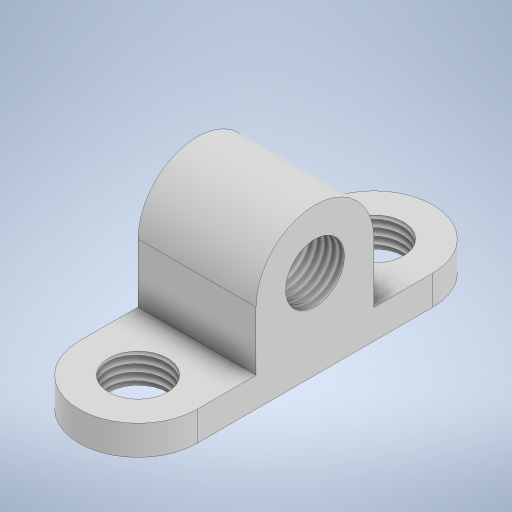
# Autodesk Inventor part: Tarea 1 Lab Dinamica
Saved by Autodesk Inventor 2024 (Build 280153000, 153)
## iProperties
Created: 2024-01-23
Part Number: Tarea 1 Lab Dinamica
Material: Genérico
Document SubType Name: Modeling
Designer: pazjo
Density: 1 g/cm^3
Appearance: Valor por defecto
Author: pazjo
Autodesk Inventor part; units mm, degrees
ref_plane "YZ Plane" through (0, 0, 0) normal (1, 0, 0) x (0, 1, 0)
ref_plane "XZ Plane" through (0, 0, 0) normal (0, 1, 0) x (-1, 0, 0)
ref_plane "XY Plane" through (0, 0, 0) normal (0, 0, 1) x (1, 0, 0)
sketch "Boceto1" plane through (0, 0, 0) normal (0, 1, 0) x (-1, 0, 0)
  line L0 (-20, 20) -> (-20, -20)
  line L1 (20, -20) -> (20, 20)
  arc A0 (20, 40) -> (-20, 40) centre (0, 40) ccw
  arc A1 (-20, -40) -> (20, -40) centre (0, -40) ccw
  circle A2 centre (0, -40) radius 10
  line L2 (20, 20) -> (20, 40)
  line L3 (-20, 20) -> (-20, 40)
  line L4 (20, -20) -> (20, -40)
  line L5 (-20, -20) -> (-20, -40)
  circle A3 centre (0, 40) radius 10
  point P0 (0, 0)
  constraints: 12 end point, 4 centre point, 4 point on circle, 3 tangent, 1 coincident, 1 parallel, 1 point on line
extrude "Extrusión1" add sketch "Boceto1" along normal blind 10
sketch "Boceto2" plane through (20, 0, 40) normal (1, 0, 0) x (0, 0, -1)
  line L0 (80, 10) -> (0, 10) construction
  circle A0 centre (40, 30) radius 10
  arc A1 (60, 30) -> (20, 30) centre (40, 30) ccw
  line L1 (20, 30) -> (20, 10)
  line L2 (60, 30) -> (60, 10)
  line L3 (20, 10) -> (60, 10)
  point P0 (40, 0)
  constraints: 6 end point, 2 centre point, 2 perpendicular, 2 point on circle, 2 point on line, 2 tangent, 1 coincident, 1 collinear
extrude "Extrusión2" add sketch "Boceto2" against normal blind 40
thread "Rosca1" size "M20x2.5" class "6H" standard "ANSI Metric M Profile" full length
thread "Rosca2" size "M20x2.5" class "6H" standard "ANSI Metric M Profile" full length
thread "Rosca3" size "M20x2.5" class "6H" standard "ANSI Metric M Profile" full length
